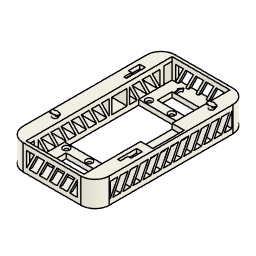
Aruba_205H_wall_support (Autodesk Fusion 360 design; units mm, degrees)
Autodesk Fusion 360 part; units mm, degrees
note: some values were not read from the file. Set by a fixed rule: which sketch regions a step uses; which face or edge a step refers to.
sketch "Boceto1" plane through (0, 0, 0) normal (0, 0, 1) x (1, 0, 0)
  line L0 (14, 0) -> (71, 0)
  line L1 (85, 14) -> (85, 136)
  line L2 (71, 150) -> (14, 150)
  line L3 (0, 136) -> (0, 14)
  arc A0 (14, 150) -> (0, 136) centre (14, 136) ccw
  arc A1 (85, 136) -> (71, 150) centre (71, 136) ccw
  arc A2 (0, 14) -> (14, 0) centre (14, 14) ccw
  arc A3 (71, 0) -> (85, 14) centre (71, 14) ccw
  line L4 (14, 150) -> (14, 0)
  line L5 (71, 150) -> (71, 0)
  point P0 (85, 0)
  point P1 (0, 150)
  dimension "d1" = 85
  dimension "d2" = 150
  dimension "d3" = 14
  dimension "d4" = 14
  dimension "d5" = 14
  dimension "d6" = 14
  constraint horizontal L0
  constraint vertical L1
  constraint horizontal L2
  constraint vertical L3
  constraint coincident P1 L3
  constraint coincident P1 L2
  constraint tangent L3 A0
  constraint tangent L2 A0
  constraint tangent L1 A1
  constraint tangent L2 A1
  constraint coincident origin L3
  constraint coincident origin L0
  constraint tangent L3 A2
  constraint tangent L0 A2
  constraint coincident P0 L1
  constraint coincident P0 L0
  constraint tangent L1 A3
  constraint tangent L0 A3
  measures "d1" distance of origin P0
  measures "d2" distance of origin P1
  measures "d3" radius of A0
  measures "d4" radius of A1
  measures "d5" radius of A2
  measures "d6" radius of A3
extrude "Extruir1" add sketch "Boceto1" along normal blind 5
sketch "Boceto2" plane through (0, 0, 5) normal (0, 0, 1) x (-1, 0, 0)
  arc A0 (-71, 0) -> (-85, -14) centre (-71, -14) ccw
  line L0 (-85, -14) -> (-85, -136)
  arc A1 (-85, -136) -> (-71, -150) centre (-71, -136) ccw
  line L1 (-71, -150) -> (-14, -150)
  arc A2 (-14, -150) -> (0, -136) centre (-14, -136) ccw
  line L2 (0, -136) -> (0, -14)
  arc A3 (0, -14) -> (-14, 0) centre (-14, -14) ccw
  line L3 (-14, 0) -> (-71, 0)
  line L4 (-14, 0) -> (-14, -150)
  line L5 (-71, -150) -> (-71, 0)
  line L6 (-14, 0) -> (-14, -3) construction
  line L7 (-14, -3) -> (-71, -3)
  line L8 (-14, -150) -> (-14, -147) construction
  line L9 (-14, -147) -> (-71, -147)
  dimension "d9" = 3
  dimension "d10" = 3
  constraint coincident A3.end L3.start
  constraint coincident L1.end A2.start
  constraint coincident A1.end L1.start
  constraint coincident A0.start L3.end
  constraint perpendicular L3 L6
  constraint coincident L5 L7.end
  constraint perpendicular L5 L7
  constraint perpendicular L1 L8
  constraint coincident L5 L9.end
  constraint perpendicular L5 L9
  measures "d9" distance of A3.end L6.end
  measures "d10" distance of L1.end L8.end
extrude "Extruir2" add sketch "Boceto2" along normal blind 20 contours A0 L0 A1 L5 | L3 L4 L5 L7 | A2 L2 A3 L4 | L1 L4 L5 L9
sketch "Boceto3" plane through (0, 0, 5) normal (0, 0, 1) x (-1, 0, 0)
  line L0 (-71, -3) -> (-71, -147)
  line L1 (-71, -147) -> (-14, -147)
  line L2 (-14, -147) -> (-14, -3)
  line L3 (-14, -3) -> (-71, -3)
  line L4 (-24, -13) -> (-61, -13)
  line L5 (-61, -13) -> (-61, -137)
  line L6 (-61, -137) -> (-24, -137)
  line L7 (-24, -137) -> (-24, -13)
  line L8 (-24, -137) -> (-24, -114) construction
  line L9 (-24, -114) -> (-61, -114)
  line L10 (-61, -13) -> (-61, -41) construction
  line L11 (-61, -41) -> (-24, -41)
  line L12 (-24, -137) -> (-24, -122.5) construction
  line L13 (-24, -122.5) -> (-61, -122.5)
  line L14 (-61, -13) -> (-61, -32.5) construction
  line L15 (-61, -32.5) -> (-24, -32.5)
  line L16 (-24, -114) -> (-14, -114)
  line L17 (-61, -114) -> (-71, -114)
  line L18 (-61, -41) -> (-71, -41)
  line L19 (-24, -41) -> (-14, -41)
  dimension "d13" = -10
  dimension "d166" = 23
  dimension "d167" = 28
  dimension "d168" = 14.5
  dimension "d169" = 19.5
  constraint perpendicular L6 L8
  constraint coincident L5 L9.end
  constraint perpendicular L5 L9
  constraint perpendicular L3 L10
  constraint coincident L7 L11.end
  constraint perpendicular L7 L11
  constraint perpendicular L6 L12
  constraint coincident L5 L13.end
  constraint perpendicular L5 L13
  constraint perpendicular L4 L14
  constraint coincident L7 L15.end
  constraint perpendicular L7 L15
  constraint coincident L2 L16.end
  constraint perpendicular L2 L16
  constraint coincident L0 L17.end
  constraint perpendicular L0 L17
  constraint coincident L0 L18.end
  constraint perpendicular L0 L18
  constraint coincident L2 L19.end
  constraint perpendicular L2 L19
  measures "d166" distance of L6.end L8.end
  measures "d167" distance of L4.end L10.end
  measures "d168" distance of L6.end L12.end
  measures "d169" distance of L4.end L14.end
extrude "Extruir3" cut sketch "Boceto3" against normal blind 30 contours L0 L5 L17 L18 | L5 L7 L9 L11 | L2 L7 L16 L19 | L4 L5 L7 L15 | L5 L6 L7 L13
sketch "Boceto4" plane through (0, 0, 5) normal (0, 0, 1) x (-1, 0, 0)
  line L0 (-71, -114) -> (-71, -147)
  line L1 (-71, -147) -> (-14, -147)
  line L2 (-14, -147) -> (-14, -114)
  line L3 (-14, -3) -> (-71, -3)
  line L4 (-26.75, -142) -> (-26.75, -146) construction
  line L5 (-25.5, -138) -> (-25.5, -142)
  line L6 (-28, -138) -> (-28, -142)
  line L7 (-26.75, -146) -> (-24, -142)
  line L8 (-25.5, -142) -> (-28, -142) construction
  line L9 (-26.75, -146) -> (-29.5, -142)
  line L10 (-25.5, -138) -> (-28, -138)
  line L11 (-28, -142) -> (-29.5, -142)
  line L12 (-25.5, -142) -> (-24, -142)
  line L13 (-24, -137) -> (-25.5, -137) construction
  line L14 (-14, -41) -> (-14, -3)
  line L15 (-71, -3) -> (-71, -41)
  point P0 (-24, -137)
  dimension "d174" = 2.5
  dimension "d175" = 4
  dimension "d176" = 4
  dimension "d177" = 1.5
  dimension "d178" = 1.5
  dimension "d179" = 4
  dimension "d205" = 5
  dimension "d206" = 1
  dimension "d207" = 1.5
  constraint perpendicular L6 L10
  constraint perpendicular L5 L10
  constraint perpendicular L5 L12
  constraint perpendicular L6 L11
  constraint midpoint L4.start L8
  constraint perpendicular L4 L8
  constraint coincident P0 L13.start
  constraint parallel L10 L13
  measures "d174" distance of L5.start L6.start
  measures "d175" distance of L6.end L6.start
  measures "d176" distance of L5.end L5.start
  measures "d177" distance of L5.end L7.end
  measures "d178" distance of L9.end L6.end
  measures "d179" distance of L4.end L4.start
  measures "d205" vertical distance of L7.end P0
  measures "d206" distance of L5.start L13.end
  measures "d207" distance of P0 L13.end
extrude "Extrude17" cut sketch "Boceto4" against normal blind 0.5
sketch "Boceto5" plane through (0, 0, 25) normal (0, 0, 1) x (-1, 0, 0)
  line L0 (-71, -3) -> (-14, -3)
  line L1 (-14, -3) -> (-14, -147)
  line L2 (-14, -147) -> (-71, -147)
  line L3 (-71, -147) -> (-71, -3)
  line L4 (-14, 0) -> (-71, 0)
  arc A0 (-71, 0) -> (-85, -14) centre (-71, -14) ccw
  line L5 (-85, -14) -> (-85, -136)
  arc A1 (-85, -136) -> (-71, -150) centre (-71, -136) ccw
  line L6 (-71, -150) -> (-14, -150)
  arc A2 (-14, -150) -> (0, -136) centre (-14, -136) ccw
  line L7 (0, -136) -> (0, -14)
  arc A3 (0, -14) -> (-14, 0) centre (-14, -14) ccw
  line L8 (0, 0) -> (0, -38) construction
  line L9 (0, -38) -> (-7.5, -38) construction
  circle A4 centre (-7.5, -38) radius 2.5
  line L10 (-71, -147) -> (-71, -122.5) construction
  line L11 (-71, -122.5) -> (-77.5, -122.5) construction
  circle A5 centre (-77.5, -122.5) radius 2.5
  line L12 (-71, -3) -> (-71, -51) construction
  line L13 (-71, -51) -> (-75, -51) construction
  line L14 (-75, -51) -> (-80.5, -51)
  line L15 (-75, -51) -> (-75, -32.5)
  line L16 (-75, -32.5) -> (-80.5, -32.5)
  line L17 (-80.5, -32.5) -> (-80.5, -51)
  line L18 (-75, -32.5) -> (-77.5, -32.5)
  line L19 (-77.5, -32.5) -> (-77.5, -40)
  line L20 (-77.5, -40) -> (-80.5, -40)
  line L21 (-14, -147) -> (-14, -106) construction
  line L22 (-14, -106) -> (-10, -106) construction
  line L23 (-4.5, -106) -> (-4.5, -124.5)
  line L24 (-4.5, -124.5) -> (-10, -124.5)
  line L25 (-10, -106) -> (-10, -124.5)
  line L26 (-4.5, -106) -> (-10, -106)
  line L27 (-4.5, -106) -> (-7.5, -106)
  line L28 (-7.5, -106) -> (-7.5, -113.5)
  line L29 (-7.5, -113.5) -> (-4.5, -113.5)
  line L30 (-4.5, -113.5) -> (-4.5, -106)
  dimension "d22" = 38
  dimension "d23" = 7.5
  dimension "d24" = 5
  dimension "d85" = 24.5
  dimension "d86" = 6.5
  dimension "d87" = 5
  dimension "d188" = 48
  dimension "d189" = 4
  dimension "d190" = 5.5
  dimension "d191" = 18.5
  dimension "d192" = 18.5
  dimension "d194" = 7.5
  dimension "d208" = 41
  dimension "d209" = 4
  dimension "d210" = 5.5
  dimension "d211" = 18.5
  dimension "d214" = 3
  dimension "d215" = 7.5
  dimension "d243" = 3
  constraint coincident L8.start origin
  constraint parallel L7 L8
  constraint perpendicular L7 L9
  constraint coincident L9.end A4.centre
  constraint coincident L2.end L3.start
  constraint perpendicular L2 L10
  constraint perpendicular L3 L11
  constraint coincident L11.end A5.centre
  constraint coincident L0.start L3.end
  constraint perpendicular L0 L12
  constraint perpendicular L3 L13
  constraint parallel L13 L14
  constraint perpendicular L13 L15
  constraint perpendicular L15 L16
  constraint perpendicular L15 L18
  constraint perpendicular L16 L19
  constraint coincident L17 L20.end
  constraint perpendicular L17 L20
  constraint coincident L1.end L2.start
  constraint perpendicular L2 L21
  constraint perpendicular L21 L22
  constraint vertical L23
  constraint horizontal L24
  constraint perpendicular L24 L25
  constraint perpendicular L25 L26
  constraint horizontal L27
  constraint vertical L28
  constraint horizontal L29
  constraint vertical L30
  measures "d22" distance of L8.start L8.end
  measures "d23" distance of L8.end L9.end
  measures "d24" diameter of A4
  measures "d85" distance of L2.end L10.end
  measures "d86" distance of L10.end L11.end
  measures "d87" diameter of A5
  measures "d188" distance of L0.start L12.end
  measures "d189" distance of L12.end L13.end
  measures "d190" distance of L13.end L14.end
  measures "d191" distance of L13.end L15.end
  measures "d192" distance of L14.end L16.end
  measures "d194" distance of L18.end L19.end
  measures "d208" distance of L1.end L21.end
  measures "d209" distance of L21.end L22.end
  measures "d210" distance of L22.end L23.start
  measures "d211" distance of L22.end L24.end
  measures "d214" distance of L23.start L27.end
  measures "d215" distance of L23.start L29.end
  measures "d243" distance of L16.end L18.end
extrude "Extruir5" add sketch "Boceto5" along normal blind 2.5 contours A4 | A5
extrude "Extrude18" cut sketch "Boceto5" against normal blind 4 contours L14 L15 L16 L17 L18 L19 L20 | L16 L17 L19 L20 | L23 L26 L27 L28 L29 L30 | L23 L24 L25 L26 L28 L29
extrude "Extrude19" add sketch "Boceto5" against normal blind 2 contours L16 L17 L19 L20 | L23 L26 L27 L28 L29 L30
sketch "Boceto6" plane through (0, 0, 0) normal (0, -1, 0) x (1, 0, 0)
  line L0 (14, 0) -> (71, 0)
  line L1 (71, 0) -> (71, 25)
  line L2 (71, 25) -> (14, 25)
  line L3 (14, 25) -> (14, 0)
  line L4 (14, 25) -> (17.5, 25) construction
  line L5 (17.5, 25) -> (17.5, 20) construction
  line L6 (17.5, 20) -> (17.5, 5)
  line L7 (17.5, 20) -> (25, 20)
  line L8 (25, 20) -> (17.5, 5)
  line L9 (25, 20) -> (27.5, 20) construction
  line L10 (27.5, 20) -> (27.5, 5)
  line L11 (27.5, 5) -> (20, 5)
  line L12 (20, 5) -> (27.5, 20)
  dimension "d30" = 3.5
  dimension "d31" = 5
  dimension "d32" = 15
  dimension "d33" = 7.5
  dimension "d34" = 2.5
  dimension "d71" = 15
  dimension "d72" = 7.5
  constraint coincident L2.end L3.start
  constraint perpendicular L1 L4
  constraint perpendicular L2 L5
  constraint perpendicular L2 L6
  constraint perpendicular L6 L7
  constraint parallel L7 L9
  constraint perpendicular L9 L10
  constraint perpendicular L10 L11
  measures "d30" distance of L2.end L4.end
  measures "d31" distance of L4.end L5.end
  measures "d32" distance of L5.end L6.end
  measures "d33" distance of L5.end L7.end
  measures "d34" distance of L7.end L9.end
  measures "d71" distance of L9.end L10.end
  measures "d72" distance of L10.end L11.end
extrude "Extruir8" add sketch "Boceto6" along normal blind 1 contours L6 L7 L8 | L10 L11 L12
pattern_linear "Patrón R2" count 5 spacing 10 along (1, 0, 0) of "Extruir8"
extrude "Extrude12" cut 6 faces at (20, -1, 15) (25, -1, 10) (35, -1, 10) (45, -1, 10) (55, -1, 10) (65, -1, 10) along direction (0, 1, 0) blind 151
sketch "Vent R" plane through (85, 0, 0) normal (1, 0, 0) x (0, 1, 0)
  line L0 (14, 0) -> (136, 0)
  line L1 (136, 0) -> (136, 25)
  line L2 (136, 25) -> (14, 25)
  line L3 (25, 5) -> (17.5, 5)
  line L4 (15, 20) -> (22.5, 20)
  line L5 (15, 20) -> (15, 5)
  line L6 (25, 20) -> (25, 5)
  line L7 (22.5, 20) -> (15, 5)
  line L8 (17.5, 5) -> (25, 20)
  line L9 (22.5, 20) -> (25, 20) construction
  line L10 (14, 0) -> (14, 25) construction
  line L11 (25, 20) -> (25, 5)
  line L12 (32.5, 20) -> (25, 5)
  line L13 (25, 20) -> (32.5, 20)
  line L14 (27.5, 5) -> (35, 20)
  line L15 (35, 20) -> (35, 5)
  line L16 (35, 5) -> (27.5, 5)
  line L17 (35, 20) -> (35, 5)
  line L18 (42.5, 20) -> (35, 5)
  line L19 (35, 20) -> (42.5, 20)
  line L20 (37.5, 5) -> (45, 20)
  line L21 (45, 20) -> (45, 5)
  line L22 (45, 5) -> (37.5, 5)
  line L23 (45, 20) -> (45, 5)
  line L24 (52.5, 20) -> (45, 5)
  line L25 (45, 20) -> (52.5, 20)
  line L26 (47.5, 5) -> (55, 20)
  line L27 (55, 20) -> (55, 5)
  line L28 (55, 5) -> (47.5, 5)
  line L29 (55, 20) -> (55, 5)
  line L30 (62.5, 20) -> (55, 5)
  line L31 (55, 20) -> (62.5, 20)
  line L32 (57.5, 5) -> (65, 20)
  line L33 (65, 20) -> (65, 5)
  line L34 (65, 5) -> (57.5, 5)
  line L35 (65, 20) -> (65, 5)
  line L36 (72.5, 20) -> (65, 5)
  line L37 (65, 20) -> (72.5, 20)
  line L38 (67.5, 5) -> (75, 20)
  line L39 (75, 20) -> (75, 5)
  line L40 (75, 5) -> (67.5, 5)
  line L41 (75, 20) -> (75, 5)
  line L42 (82.5, 20) -> (75, 5)
  line L43 (75, 20) -> (82.5, 20)
  line L44 (77.5, 5) -> (85, 20)
  line L45 (85, 20) -> (85, 5)
  line L46 (85, 5) -> (77.5, 5)
  line L47 (85, 20) -> (85, 5)
  line L48 (92.5, 20) -> (85, 5)
  line L49 (85, 20) -> (92.5, 20)
  line L50 (87.5, 5) -> (95, 20)
  line L51 (95, 20) -> (95, 5)
  line L52 (95, 5) -> (87.5, 5)
  line L53 (95, 20) -> (95, 5)
  line L54 (102.5, 20) -> (95, 5)
  line L55 (95, 20) -> (102.5, 20)
  line L56 (97.5, 5) -> (105, 20)
  line L57 (105, 20) -> (105, 5)
  line L58 (105, 5) -> (97.5, 5)
  line L59 (105, 20) -> (105, 5)
  line L60 (112.5, 20) -> (105, 5)
  line L61 (105, 20) -> (112.5, 20)
  line L62 (107.5, 5) -> (115, 20)
  line L63 (115, 20) -> (115, 5)
  line L64 (115, 5) -> (107.5, 5)
  line L65 (115, 20) -> (115, 5)
  line L66 (122.5, 20) -> (115, 5)
  line L67 (115, 20) -> (122.5, 20)
  line L68 (117.5, 5) -> (125, 20)
  line L69 (125, 20) -> (125, 5)
  line L70 (125, 5) -> (117.5, 5)
  line L71 (125, 20) -> (125, 5)
  line L72 (132.5, 20) -> (125, 5)
  line L73 (125, 20) -> (132.5, 20)
  line L74 (127.5, 5) -> (135, 20)
  line L75 (135, 20) -> (135, 5)
  line L76 (135, 5) -> (127.5, 5)
  dimension "d91" = 15
  dimension "d92" = 7.5
  dimension "d93" = 2.5
  dimension "d94" = 15
  dimension "d95" = 7.5
  dimension "d100" = 5
  dimension "d101" = 1
  dimension "d102" = 1
  dimension "d105" = 110
  dimension "d106" = 0
  constraint perpendicular L4 L5
  constraint parallel L4 L9
  constraint perpendicular L6 L9
  constraint perpendicular L3 L6
  measures "d91" distance of L5.end L4.start
  measures "d92" distance of L4.end L4.start
  measures "d93" distance of L4.end L6.start
  measures "d94" distance of L6.start L3.start
  measures "d95" distance of L3.end L3.start
  measures "d100" distance of L2 L4.start
  measures "d101" distance of L5.end L10
  measures "d102" distance of L4.start L10
extrude "Extrude13" cut sketch "Vent R" against normal blind 24
sketch "Vent L" plane through (0, 0, 0) normal (-1, 0, 0) x (0, -1, 0)
  line L0 (-136, 0) -> (-14, 0)
  line L1 (-14, 0) -> (-14, 25)
  line L2 (-14, 25) -> (-136, 25)
  line L3 (-136, 25) -> (-136, 0)
  line L4 (-125, 5) -> (-132.5, 5)
  line L5 (-135, 20) -> (-135, 5)
  line L6 (-125, 20) -> (-125, 5)
  line L7 (-127.5, 20) -> (-135, 5)
  line L8 (-132.5, 5) -> (-125, 20)
  line L9 (-127.5, 20) -> (-125, 20) construction
  line L10 (-135, 20) -> (-127.5, 20)
  line L11 (-132.5, 5) -> (-135, 5) construction
  line L12 (-125, 20) -> (-125, 5)
  line L13 (-117.5, 20) -> (-125, 5)
  line L14 (-125, 20) -> (-117.5, 20)
  line L15 (-115, 20) -> (-115, 5)
  line L16 (-122.5, 5) -> (-115, 20)
  line L17 (-115, 5) -> (-122.5, 5)
  line L18 (-115, 20) -> (-115, 5)
  line L19 (-107.5, 20) -> (-115, 5)
  line L20 (-115, 20) -> (-107.5, 20)
  line L21 (-105, 20) -> (-105, 5)
  line L22 (-112.5, 5) -> (-105, 20)
  line L23 (-105, 5) -> (-112.5, 5)
  line L24 (-105, 20) -> (-105, 5)
  line L25 (-97.5, 20) -> (-105, 5)
  line L26 (-105, 20) -> (-97.5, 20)
  line L27 (-95, 20) -> (-95, 5)
  line L28 (-102.5, 5) -> (-95, 20)
  line L29 (-95, 5) -> (-102.5, 5)
  line L30 (-95, 20) -> (-95, 5)
  line L31 (-87.5, 20) -> (-95, 5)
  line L32 (-95, 20) -> (-87.5, 20)
  line L33 (-85, 20) -> (-85, 5)
  line L34 (-92.5, 5) -> (-85, 20)
  line L35 (-85, 5) -> (-92.5, 5)
  line L36 (-85, 20) -> (-85, 5)
  line L37 (-77.5, 20) -> (-85, 5)
  line L38 (-85, 20) -> (-77.5, 20)
  line L39 (-75, 20) -> (-75, 5)
  line L40 (-82.5, 5) -> (-75, 20)
  line L41 (-75, 5) -> (-82.5, 5)
  line L42 (-75, 20) -> (-75, 5)
  line L43 (-67.5, 20) -> (-75, 5)
  line L44 (-75, 20) -> (-67.5, 20)
  line L45 (-65, 20) -> (-65, 5)
  line L46 (-72.5, 5) -> (-65, 20)
  line L47 (-65, 5) -> (-72.5, 5)
  line L48 (-65, 20) -> (-65, 5)
  line L49 (-57.5, 20) -> (-65, 5)
  line L50 (-65, 20) -> (-57.5, 20)
  line L51 (-55, 20) -> (-55, 5)
  line L52 (-62.5, 5) -> (-55, 20)
  line L53 (-55, 5) -> (-62.5, 5)
  line L54 (-55, 20) -> (-55, 5)
  line L55 (-47.5, 20) -> (-55, 5)
  line L56 (-55, 20) -> (-47.5, 20)
  line L57 (-45, 20) -> (-45, 5)
  line L58 (-52.5, 5) -> (-45, 20)
  line L59 (-45, 5) -> (-52.5, 5)
  line L60 (-45, 20) -> (-45, 5)
  line L61 (-37.5, 20) -> (-45, 5)
  line L62 (-45, 20) -> (-37.5, 20)
  line L63 (-35, 20) -> (-35, 5)
  line L64 (-42.5, 5) -> (-35, 20)
  line L65 (-35, 5) -> (-42.5, 5)
  line L66 (-35, 20) -> (-35, 5)
  line L67 (-27.5, 20) -> (-35, 5)
  line L68 (-35, 20) -> (-27.5, 20)
  line L69 (-25, 20) -> (-25, 5)
  line L70 (-32.5, 5) -> (-25, 20)
  line L71 (-25, 5) -> (-32.5, 5)
  line L72 (-25, 20) -> (-25, 5)
  line L73 (-17.5, 20) -> (-25, 5)
  line L74 (-25, 20) -> (-17.5, 20)
  line L75 (-15, 20) -> (-15, 5)
  line L76 (-22.5, 5) -> (-15, 20)
  line L77 (-15, 5) -> (-22.5, 5)
  dimension "d111" = 15
  dimension "d112" = 7.5
  dimension "d113" = 2.5
  dimension "d114" = 15
  dimension "d115" = 7.5
  dimension "d116" = 1
  dimension "d117" = 1
  dimension "d118" = 5
  dimension "d119" = 2.5
  dimension "d122" = 110
  dimension "d123" = 0
  constraint perpendicular L6 L9
  constraint perpendicular L4 L6
  constraint perpendicular L5 L10
  measures "d111" distance of L5.end L5.start
  measures "d112" distance of L7.start L5.start
  measures "d113" distance of L7.start L6.start
  measures "d114" distance of L6.start L4.start
  measures "d115" distance of L4.end L4.start
  measures "d116" distance of L3 L5.start
  measures "d117" distance of L3 L5.end
  measures "d118" distance of L2 L5.start
  measures "d119" distance of L5.end L4.end
extrude "Extrude14" cut sketch "Vent L" against normal blind 14 contours L4 L6 L8 L12 | L6 L12 L13 L14 | L5 L7 L10 | L15 L18 L19 L20 | L15 L16 L17 L18 | L21 L22 L23 L24 | L33 L36 L37 L38 | L39 L42 L43 L44 | L39 L40 L41 L42 | L45 L48 L49 L50 | L45 L46 L47 L48 | L51 L54 L55 L56 | L51 L52 L53 L54 | L57 L60 L61 L62 | L57 L58 L59 L60 | L63 L66 L67 L68 | L63 L64 L65 L66 | L69 L72 L73 L74 | L69 L70 L71 L72 | L75 L76 L77
sketch "Ledge 1" plane through (0, 0, 27.5) normal (0, 0, 1) x (-1, 0, 0)
  circle A0 centre (-7.5, -38) radius 2.5
  line L0 (-7.5, -38) -> (-7.5, -36.25) construction
  line L1 (-7.5, -38) -> (-7.5, -39.75) construction
  line L2 (-7.5, -39.75) -> (-11, -39.75)
  line L3 (-7.5, -36.25) -> (-11, -36.25)
  arc A1 (-11, -36.25) -> (-11, -39.75) centre (-8.687, -38) ccw
  line L4 (-7.5, -39.75) -> (-4, -39.75)
  line L5 (-7.5, -36.25) -> (-4, -36.25)
  line L6 (-7.5, -38) -> (-3.4125, -38) construction
  arc A2 (-4, -39.75) -> (-4, -36.25) centre (-6.3125, -38) ccw
  line L7 (-7.5, -38) -> (-11.5874, -38) construction
  dimension "d130" = 1.75
  dimension "d131" = 1.75
  dimension "d132" = 3.5
  dimension "d134" = 3.5
  dimension "d135" = 1.187
  dimension "d136" = 3.5
  dimension "d137" = 3.5
  dimension "d138" = 1.1875
  constraint coincident A0.centre L0.start
  constraint vertical L0
  constraint parallel L0 L1
  constraint perpendicular L1 L2
  constraint perpendicular L0 L3
  constraint perpendicular L1 L4
  constraint perpendicular L0 L5
  constraint perpendicular L1 L6
  constraint coincident L6.end A2
  constraint midpoint A1 L7.end
  measures "d130" distance of A0.centre L0.end
  measures "d131" distance of A0.centre L1.end
  measures "d132" distance of L1.end L2.end
  measures "d134" distance of L0.end L3.end
  measures "d135" distance of A0.centre A1.centre
  measures "d136" distance of L1.end L4.end
  measures "d137" distance of L0.end L5.end
  measures "d138" distance of A0.centre A2.centre
sketch "Ledge 2" plane through (0, 0, 27.5) normal (0, 0, 1) x (-1, 0, 0)
  circle A0 centre (-77.5, -122.5) radius 2.5
  line L0 (-77.5, -122.5) -> (-77.5, -124.25) construction
  line L1 (-77.5, -122.5) -> (-77.5, -120.75) construction
  line L2 (-77.5, -124.25) -> (-81, -124.25)
  line L3 (-77.5, -120.75) -> (-81, -120.75)
  line L4 (-77.5, -124.25) -> (-74, -124.25)
  line L5 (-77.5, -120.75) -> (-74, -120.75)
  line L6 (-77.5, -122.5) -> (-73.5, -122.5) construction
  arc A1 (-74, -124.25) -> (-74, -120.75) centre (-76.8125, -122.5) ccw
  line L7 (-77.5, -122.5) -> (-81.5875, -122.5) construction
  arc A2 (-81, -120.75) -> (-81, -124.25) centre (-78.6875, -122.5) ccw
  dimension "d158" = 1.75
  dimension "d159" = 1.75
  dimension "d160" = 3.5
  dimension "d161" = 3.5
  dimension "d162" = 3.5
  dimension "d163" = 3.5
  dimension "d164" = 4
  dimension "d165" = 1.1875
  constraint coincident A0.centre L0.start
  constraint vertical L0
  constraint parallel L0 L1
  constraint perpendicular L0 L2
  constraint perpendicular L1 L3
  constraint perpendicular L0 L4
  constraint perpendicular L1 L5
  constraint perpendicular L0 L6
  constraint coincident L6.end A1
  constraint perpendicular L1 L7
  constraint coincident L7.end A2
  measures "d158" distance of A0.centre L0.end
  measures "d159" distance of A0.centre L1.end
  measures "d160" distance of L0.end L2.end
  measures "d161" distance of L1.end L3.end
  measures "d162" distance of L0.end L4.end
  measures "d163" distance of L1.end L5.end
  measures "d164" distance of A0.centre L6.end
  measures "d165" distance of A0.centre A2.centre
extrude "Extrude16" add sketch "Ledge 1" sketch "Ledge 2" along normal blind 1 of sketch 2
sketch "Screw holes" plane through (0, 0, 5) normal (0, 0, 1) x (-1, 0, 0)
  line L0 (-71, -25) -> (-71, -27.5)
  line L1 (-85, -27.5) -> (-85, -35)
  line L2 (-67.5, 0) -> (-67.5, -3)
  line L3 (-60, -3) -> (-60, 0)
  line L4 (-57.5, 0) -> (-57.5, -3)
  line L5 (-50, -3) -> (-50, 0)
  line L6 (-47.5, 0) -> (-47.5, -3)
  line L7 (-40, -3) -> (-40, 0)
  line L8 (-37.5, 0) -> (-37.5, -3)
  line L9 (-30, -3) -> (-30, 0)
  line L10 (-27.5, 0) -> (-27.5, -3)
  line L11 (-20, -3) -> (-20, 0)
  line L12 (-14, -35) -> (-14, -32.5)
  line L13 (-61, -32.5) -> (-61, -13)
  line L14 (-24, -13) -> (-24, -32.5)
  circle A0 centre (-42.5, -36.75) radius 1.25
  line L15 (-42.5, -36.75) -> (-20, -36.75) construction
  line L16 (-42.5, -36.75) -> (-65, -36.75) construction
  circle A1 centre (-20, -36.75) radius 1.25
  circle A2 centre (-65, -36.75) radius 1.25
  line L17 (-42.5, -122.5) -> (-42.5, -118.25) construction
  circle A3 centre (-42.5, -118.25) radius 1.25
  line L18 (-42.5, -118.25) -> (-20, -118.25) construction
  line L19 (-42.5, -118.25) -> (-65, -118.25) construction
  circle A4 centre (-65, -118.25) radius 1.25
  circle A5 centre (-20, -118.25) radius 1.25
  line L20 (-14, -3) -> (-14, -147)
  line L21 (-14, -41) -> (-42.5, -41) construction
  line L22 (-42.5, -41) -> (-42.5, -36.75) construction
  line L23 (-71, -147) -> (-71, -3) construction
  line L24 (-71, -27.5) -> (-85, -27.5)
  line L25 (-85, -35) -> (-71, -35)
  line L26 (-71, -35) -> (-71, -37.5)
  line L27 (-71, -37.5) -> (-85, -37.5)
  line L28 (-85, -37.5) -> (-85, -45)
  line L29 (-85, -45) -> (-71, -45)
  line L30 (-71, -45) -> (-71, -41)
  line L31 (-71, -41) -> (-14, -41)
  line L32 (-14, -41) -> (-14, -35)
  line L33 (-14, -32.5) -> (-14, -25)
  line L34 (-14, -25) -> (-14, -22.5)
  line L35 (-14, -22.5) -> (-14, -15)
  line L36 (-14, -15) -> (-14, -3)
  line L37 (-14, -3) -> (-17.5, -3)
  line L38 (-17.5, -3) -> (-20, -3)
  line L39 (-20, 0) -> (-27.5, 0)
  line L40 (-27.5, -3) -> (-30, -3)
  line L41 (-30, 0) -> (-37.5, 0)
  line L42 (-37.5, -3) -> (-40, -3)
  line L43 (-40, 0) -> (-47.5, 0)
  line L44 (-47.5, -3) -> (-50, -3)
  line L45 (-50, 0) -> (-57.5, 0)
  line L46 (-57.5, -3) -> (-60, -3)
  line L47 (-60, 0) -> (-67.5, 0)
  line L48 (-67.5, -3) -> (-71, -3)
  line L49 (-71, -3) -> (-71, -15)
  line L50 (-71, -15) -> (-71, -17.5)
  line L51 (-71, -17.5) -> (-85, -17.5)
  line L52 (-85, -17.5) -> (-85, -25)
  line L53 (-85, -25) -> (-71, -25)
  line L54 (-61, -13) -> (-24, -13)
  line L55 (-24, -32.5) -> (-61, -32.5)
  line L56 (-14, -114) -> (-71, -114)
  dimension "d217" = 2.5
  dimension "d218" = 22.5
  dimension "d220" = 2.5
  dimension "d221" = 2.5
  dimension "d222" = 4.25
  dimension "d223" = 2.5
  dimension "d224" = 22.5
  dimension "d225" = 22.5
  dimension "d226" = 2.5
  dimension "d227" = 2.5
  dimension "d251" = 28.5
  dimension "d252" = 4.25
  dimension "d253" = 22.5
  dimension "d254" = 38
  dimension "d255" = 6
  dimension "d256" = 6
  dimension "d263" = 4.25
  dimension "d264" = 4.25
  dimension "d265" = 6
  constraint coincident A0.centre L15.start
  constraint coincident L15.end A1.centre
  constraint coincident L16.end A2.centre
  constraint coincident L17.end A3.centre
  constraint perpendicular L17 L18
  constraint perpendicular L17 L19
  constraint coincident L19.end A4.centre
  constraint coincident L18.end A5.centre
  constraint coincident L20 L21.start
  constraint perpendicular L20 L21
  measures "d217" diameter of A0
  measures "d218" distance of A0.centre L15.end
  measures "d220" diameter of A1
  measures "d221" diameter of A2
  measures "d222" distance of L17.start L17.end
  measures "d223" diameter of A3
  measures "d224" distance of L17.end L18.end
  measures "d225" distance of L17.end L19.end
  measures "d226" diameter of A4
  measures "d227" diameter of A5
  measures "d251" distance of L21.start L21.end
  measures "d252" distance of A0.centre L21.end
  measures "d253" distance of A0.centre L16.end
  measures "d254" distance of L20.start L21.start
  measures "d255" distance of L15.end L20
  measures "d256" distance of L16.end L23
  measures "d263" distance of L18.end L56
  measures "d264" distance of L19.end L56
  measures "d265" distance of L18.end L20
hole "Hole1" at (20, 118.25, 5) at (20, 36.75, 5) at (42.5, 36.75, 5) at (42.5, 118.25, 5) at (65, 118.25, 5) at (65, 36.75, 5) direction (0, 0, -1) diameter 3.5 depth 8 tip angle 118 countersink diameter 6.5 countersink angle 90
sketch "Fit hole" plane through (0, 0, 25) normal (0, 0, 1) x (-1, 0, 0)
  line L0 (-77.5, -32.5) -> (-75, -32.5)
  line L1 (-75, -32.5) -> (-75, -51)
  line L2 (-75, -51) -> (-80.5, -51)
  line L3 (-80.5, -51) -> (-80.5, -40)
  line L4 (-80.5, -40) -> (-77.5, -40)
  line L5 (-77.5, -40) -> (-77.5, -32.5)
  line L6 (-10, -106) -> (-7.5, -106)
  line L7 (-7.5, -106) -> (-7.5, -113.5)
  line L8 (-7.5, -113.5) -> (-4.5, -113.5)
  line L9 (-4.5, -113.5) -> (-4.5, -124.5)
  line L10 (-4.5, -124.5) -> (-10, -124.5)
  line L11 (-10, -124.5) -> (-10, -106)
  circle A0 centre (-77.5, -122.5) radius 2.5
  circle A1 centre (-7.5, -38) radius 2.5
  line L12 (-71, -3) -> (-14, -3)
  line L13 (-14, -3) -> (-14, -147)
  line L14 (-14, -147) -> (-71, -147)
  line L15 (-71, -147) -> (-71, -3)
  line L16 (-14, 0) -> (-71, 0)
  arc A2 (-71, 0) -> (-85, -14) centre (-71, -14) ccw
  line L17 (-85, -14) -> (-85, -136)
  arc A3 (-85, -136) -> (-71, -150) centre (-71, -136) ccw
  line L18 (-71, -150) -> (-14, -150)
  arc A4 (-14, -150) -> (0, -136) centre (-14, -136) ccw
  line L19 (0, -136) -> (0, -14)
  arc A5 (0, -14) -> (-14, 0) centre (-14, -14) ccw
  line L20 (-75, -51) -> (-71, -51) construction
  line L21 (-71, -51) -> (-71, -59) construction
  line L22 (-71, -59) -> (-83, -59)
  line L23 (-83, -59) -> (-83, -90)
  line L24 (-83, -90) -> (-71, -90)
  line L25 (-71, -90) -> (-71, -59)
  dimension "d234" = 8
  dimension "d235" = 12
  dimension "d236" = 31
  constraint coincident L1.end L2.start
  constraint coincident L15 L20.end
  constraint perpendicular L15 L20
  constraint perpendicular L20 L21
  constraint horizontal L22
  constraint vertical L23
  constraint horizontal L24
  constraint vertical L25
  measures "d234" distance of L20.end L21.end
  measures "d235" distance of L21.end L22.end
  measures "d236" distance of L21.end L24.end
extrude "Extrude20" cut sketch "Fit hole" against normal blind 5 contours L15 L22 L23 L24 L25
sketch "Fit hole barrier" plane through (0, 0, 20) normal (0, 0, 1) x (-1, 0, 0)
  line L0 (-83, -55) -> (-71, -55)
  line L1 (-71, -55) -> (-71, -93)
  line L2 (-71, -93) -> (-83, -93)
  line L3 (-83, -93) -> (-83, -55)
  line L4 (-85, -14) -> (-85, -136)
  line L5 (-85, -45) -> (-71, -45)
  dimension "d266" = 12
  dimension "d267" = 38
  dimension "d268" = 2
  dimension "d269" = 10
  constraint horizontal L0
  constraint vertical L1
  constraint horizontal L2
  constraint vertical L3
  measures "d266" distance of L0.start L0.end
  measures "d267" distance of L0.end L1.end
  measures "d268" distance of L0.start L4
  measures "d269" distance of L0.start L5
extrude "Extrude23" add sketch "Fit hole barrier" against normal blind 2.5
extrude "Extrude24" add 1 faces at (75, 55, 18.3333) along direction (0, -1, 0) blind 2
sketch "Material hole" plane through (0, 0, 0) normal (0, 0, -1) x (1, 0, 0)
  circle A0 centre (65, -118.25) radius 1.75
  circle A1 centre (42.5, -36.75) radius 1.75
  circle A2 centre (20, -118.25) radius 1.75
  circle A3 centre (20, -36.75) radius 1.75
  circle A4 centre (42.5, -118.25) radius 1.75
  circle A5 centre (65, -36.75) radius 1.75
  line L0 (24, -32.5) -> (24, -13)
  line L1 (24, -13) -> (61, -13)
  line L2 (61, -13) -> (61, -32.5)
  line L3 (61, -32.5) -> (24, -32.5)
  line L4 (71, -41) -> (71, -114)
  line L5 (71, -114) -> (14, -114)
  line L6 (14, -114) -> (14, -41)
  line L7 (14, -41) -> (71, -41)
  line L8 (61, -122.5) -> (61, -137)
  line L9 (61, -137) -> (24, -137)
  line L10 (24, -137) -> (24, -122.5)
  line L11 (24, -122.5) -> (61, -122.5)
  arc A6 (85, -14) -> (71, 0) centre (71, -14) ccw
  line L12 (71, 0) -> (14, 0)
  arc A7 (14, 0) -> (0, -14) centre (14, -14) ccw
  line L13 (0, -14) -> (0, -136)
  arc A8 (0, -136) -> (14, -150) centre (14, -136) ccw
  line L14 (14, -150) -> (71, -150)
  arc A9 (71, -150) -> (85, -136) centre (71, -136) ccw
  line L15 (85, -136) -> (85, -14)
  arc A10 (3, -136) -> (14, -147) centre (14, -136) ccw
  line L16 (14, -147) -> (71, -147)
  arc A11 (71, -147) -> (82, -136) centre (71, -136) ccw
  line L17 (82, -136) -> (82, -14)
  arc A12 (82, -14) -> (71, -3) centre (71, -14) ccw
  line L18 (71, -3) -> (14, -3)
  arc A13 (14, -3) -> (3, -14) centre (14, -14) ccw
  line L19 (3, -14) -> (3, -136)
  arc A14 (11, -136) -> (14, -139) centre (14, -136) ccw
  line L20 (14, -139) -> (71, -139)
  arc A15 (71, -139) -> (74, -136) centre (71, -136) ccw
  line L21 (74, -136) -> (74, -14)
  arc A16 (74, -14) -> (71, -11) centre (71, -14) ccw
  line L22 (71, -11) -> (14, -11)
  arc A17 (14, -11) -> (11, -14) centre (14, -14) ccw
  line L23 (11, -14) -> (11, -136)
  line L24 (14, -3) -> (14, -11)
  line L25 (71, -11) -> (71, -3)
  line L26 (3, -136) -> (11, -136)
  line L27 (14, -147) -> (14, -139)
  line L28 (71, -147) -> (71, -139)
  line L29 (82, -136) -> (74, -136)
  line L30 (11, -14) -> (3, -14)
  line L31 (74, -14) -> (82, -14)
  dimension "d257" = -3
  dimension "d258" = -11
  constraint perpendicular L22 L24
  constraint perpendicular L18 L25
  constraint perpendicular L23 L26
  constraint perpendicular L20 L27
  constraint perpendicular L20 L28
  constraint perpendicular L21 L29
  constraint perpendicular L19 L30
  constraint perpendicular L17 L31
extrude "Extrude22" cut sketch "Material hole" against normal blind 21 contours A10 A14 L26 L27 | A13 A17 L24 L30 | A11 A15 L28 L29 | A12 A16 L25 L31
sketch "Sketch20" plane through (0, 0, 0) normal (-1, 0, 0) x (0, -1, 0)
  line L0 (-25, 5) -> (-32.5, 5)
  line L1 (-32.5, 5) -> (-25, 20)
  line L2 (-25, 20) -> (-17.5, 20)
  line L3 (-17.5, 20) -> (-25, 5)
  line L4 (-65, 5) -> (-72.5, 5)
  line L5 (-72.5, 5) -> (-65, 20)
  line L6 (-65, 20) -> (-57.5, 20)
  line L7 (-57.5, 20) -> (-65, 5)
  line L8 (-125, 5) -> (-132.5, 5)
  line L9 (-132.5, 5) -> (-125, 20)
  line L10 (-125, 20) -> (-117.5, 20)
  line L11 (-117.5, 20) -> (-125, 5)
  line L12 (-115, 5) -> (-122.5, 5)
  line L13 (-122.5, 5) -> (-115, 20)
  line L14 (-115, 20) -> (-107.5, 20)
  line L15 (-107.5, 20) -> (-115, 5)
  line L16 (-55, 5) -> (-62.5, 5)
  line L17 (-62.5, 5) -> (-55, 20)
  line L18 (-55, 20) -> (-47.5, 20)
  line L19 (-47.5, 20) -> (-55, 5)
  line L20 (-22.5, 5) -> (-15, 20)
  line L21 (-15, 20) -> (-15, 5)
  line L22 (-15, 5) -> (-22.5, 5)
  line L23 (-35, 5) -> (-42.5, 5)
  line L24 (-42.5, 5) -> (-35, 20)
  line L25 (-35, 20) -> (-27.5, 20)
  line L26 (-27.5, 20) -> (-35, 5)
  line L27 (-75, 5) -> (-82.5, 5)
  line L28 (-82.5, 5) -> (-75, 20)
  line L29 (-75, 20) -> (-67.5, 20)
  line L30 (-67.5, 20) -> (-75, 5)
  line L31 (-127.5, 20) -> (-135, 5)
  line L32 (-135, 5) -> (-135, 20)
  line L33 (-135, 20) -> (-127.5, 20)
  line L34 (-105, 5) -> (-112.5, 5)
  line L35 (-112.5, 5) -> (-105, 20)
  line L36 (-105, 20) -> (-105, 5)
  line L37 (-45, 5) -> (-52.5, 5)
  line L38 (-52.5, 5) -> (-45, 20)
  line L39 (-45, 20) -> (-37.5, 20)
  line L40 (-37.5, 20) -> (-45, 5)
  line L41 (-77.5, 20) -> (-85, 5)
  line L42 (-85, 5) -> (-85, 20)
  line L43 (-85, 20) -> (-77.5, 20)
  line L44 (-136, 0) -> (-14, 0)
  line L45 (-14, 0) -> (-14, 25)
  line L46 (-14, 25) -> (-136, 25)
  line L47 (-136, 25) -> (-136, 0)
  line L48 (-102.5, 5) -> (-87.5, 5)
  line L49 (-87.5, 5) -> (-87.5, 20)
  line L50 (-87.5, 20) -> (-102.5, 20)
  line L51 (-102.5, 20) -> (-102.5, 5)
  dimension "d274" = 15
  dimension "d275" = 15
  dimension "d276" = 2.5
  dimension "d277" = 5
  constraint horizontal L48
  constraint vertical L49
  constraint horizontal L50
  constraint vertical L51
  measures "d274" distance of L48.start L48.end
  measures "d275" distance of L48.start L50.end
  measures "d276" distance of L36 L51
  measures "d277" distance of L44 L48
extrude "Extrude25" cut sketch "Sketch20" against normal blind 14 contours L48 L49 L50 L51
